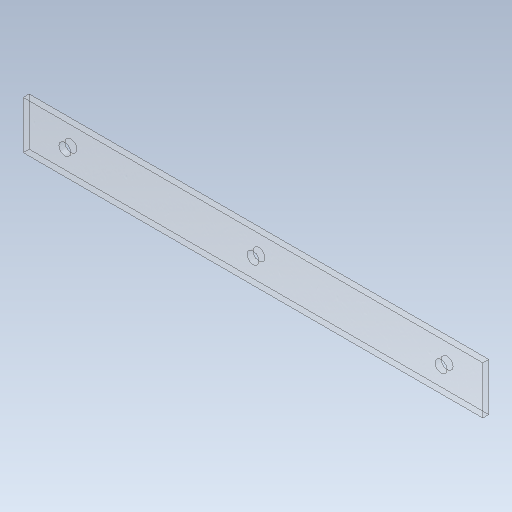
# Autodesk Inventor part: Sup.Acrilico.Segur
Saved by Autodesk Inventor 2020 (Build 240168000, 168)
## iProperties
Created: 2018-06-05
Part Number: Sup.Acrilico.Segur
Material: Acrílico, claro
Document SubType Name: Modeling
Designer: Cristiano
Density: 1.19 g/cm^3
Appearance: Transparente - Claro
Mass: 231.737 g
Surface Area: 494.243 cm^2
Volume: 304.917 cm^3
Author: Cristiano
Autodesk Inventor part; units mm, degrees
ref_plane "YZ Plane" through (0, 0, 0) normal (1, 0, 0) x (0, 1, 0)
ref_plane "XZ Plane" through (0, 0, 0) normal (0, 1, 0) x (-1, 0, 0)
ref_plane "XY Plane" through (0, 0, 0) normal (0, 0, 1) x (1, 0, 0)
sketch "Boceto1" plane through (0, 0, 0) normal (0, 0, 1) x (1, 0, 0)
  line L0 (0, 0) -> (385, 0)
  line L1 (385, 0) -> (385, 40)
  line L2 (385, 40) -> (0, 40)
  line L3 (0, 40) -> (0, 0)
  line L4 (0, 20) -> (385, 20) construction
  circle A0 centre (35, 20) radius 5
  circle A1 centre (192.5, 20) radius 5
  circle A2 centre (350, 20) radius 5
  dimension "d0" = 40
  dimension "d1" = 385
  dimension "d2" = 10
  dimension "d3" = 10
  dimension "d4" = 10
  dimension "d5" = 35
  dimension "d6" = 35
  constraints: 10 end point, 3 centre point, 3 midpoint, 2 parallel, 2 point on line, 1 horizontal, 1 perpendicular
  measures "d0" distance of L2.end L0.start
  measures "d1" distance of L0.start L0.end
  measures "d2" diameter of A0
  measures "d3" diameter of A1
  measures "d4" diameter of A2
  measures "d5" distance of L4.start A0.centre
  measures "d6" distance from line of L1 A2.centre
extrude "Extrusión1" add sketch "Boceto1" along normal blind 5
